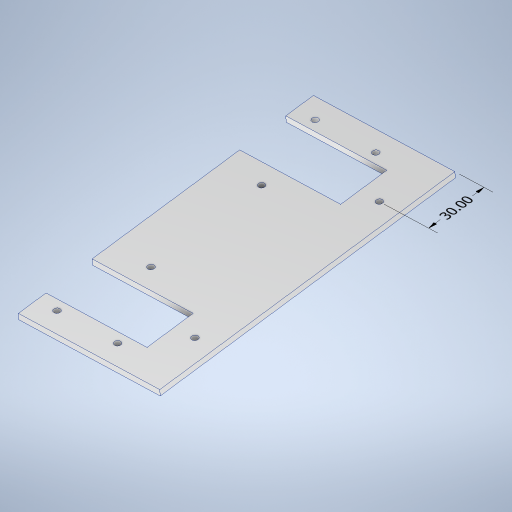
# Autodesk Inventor part: backPlate
Saved by Autodesk Inventor 2024 (Build 280153000, 153)
## iProperties
Created: 2023-10-26
Part Number: backPlate
Material: アルミニウム 6061
Document SubType Name: Modeling
Designer: jwith
Density: 2.7 g/cm^3
Appearance: アルミニウム - フラット
Mass: 69.9488 g
Surface Area: 194.926 cm^2
Volume: 25.907 cm^3
Author: jwith
Autodesk Inventor part; units mm, degrees
ref_plane "YZ Plane" through (0, 0, 0) normal (1, 0, 0) x (0, 1, 0)
ref_plane "XZ Plane" through (0, 0, 0) normal (0, 1, 0) x (-1, 0, 0)
ref_plane "XY Plane" through (0, 0, 0) normal (0, 0, 1) x (1, 0, 0)
sketch "スケッチ1" plane through (0, 0, 0) normal (0, 0, 1) x (1, 0, 0)
  line L0 (0, 0) -> (160, 0)
  line L1 (160, 0) -> (160, 70)
  line L2 (160, 70) -> (0, 70)
  line L3 (0, 70) -> (0, 0)
  line L4 (20, 0) -> (40, 0)
  line L5 (40, 0) -> (40, 50)
  line L6 (40, 50) -> (20, 50)
  line L7 (20, 50) -> (20, 0)
  line L8 (140, 0) -> (120, 0)
  line L9 (120, 0) -> (120, 50)
  line L10 (120, 50) -> (140, 50)
  line L11 (140, 50) -> (140, 0)
  dimension "d0" = 70
  dimension "d1" = 160
  dimension "d2" = 20
  dimension "d3" = 20
  dimension "d4" = 50
  dimension "d5" = 20
  dimension "d6" = 20
  dimension "d7" = 50
  constraints: 24 end point, 6 parallel, 3 horizontal, 3 perpendicular, 2 point on line
  measures "d0" distance of L0.end L1.end
  measures "d1" distance of L1.end L2.end
  measures "d2" distance between parallel lines of L3 L7
  measures "d3" distance of L5.end L6.end
  measures "d4" distance of L4.end L5.end
  measures "d5" distance between parallel lines of L1 L11
  measures "d6" distance of L9.end L10.end
  measures "d7" distance of L10.end L8.start
extrude "押し出し1" add sketch "スケッチ1" along normal blind 3 contours L3 L2 L1 L0 L11 L10 L9 L5 L6 L7
sketch "スケッチ2" plane through (0, 0, 3) normal (0, 0, 1) x (1, 0, 0)
  line L0 (0, 70) -> (0, 0) projected
  line L1 (0, 0) -> (20, 0) projected
  line L2 (140, 0) -> (160, 0) projected
  line L3 (160, 0) -> (160, 70) projected
  point P0 (10, 10)
  point P1 (150, 10)
  point P2 (10, 40)
  point P3 (150, 40)
  dimension "d10" = 10
  dimension "d11" = 10
  dimension "d12" = 10
  dimension "d13" = 10
  dimension "d14" = 30
  dimension "d15" = 10
  dimension "d16" = 10
  dimension "d17" = 30
  measures "d10" distance from line of L0 point (10, 10)
  measures "d11" distance from line of L1 point (10, 10)
  measures "d12" distance from line of L2 point (150, 10)
  measures "d13" distance from line of L3 point (150, 10)
  measures "d14" distance of point (10, 10) point (10, 40)
  measures "d15" distance from line of L0 point (10, 40)
  measures "d16" distance from line of L3 point (150, 40)
  measures "d17" distance of point (150, 10) point (150, 40)
hole "穴1" at (10, 10, 3) at (150, 10, 3) at (10, 40, 3) at (150, 40, 3) direction (0, 0, -1) diameter 3.2 end through all
sketch "スケッチ3" plane through (0, 0, 3) normal (0, 0, 1) x (1, 0, 0)
  line L0 (0, 70) -> (0, 0) projected
  line L1 (160, 70) -> (0, 70) projected
  point P0 (30, 60)
  point P1 (130, 60)
  dimension "d25" = 30
  dimension "d26" = 10
  dimension "d27" = 10
  dimension "d28" = 100
  measures "d25" distance from line of L0 point (30, 60)
  measures "d26" distance from line of L1 point (30, 60)
  measures "d27" distance from line of L1 point (130, 60)
  measures "d28" distance of point (130, 60) point (30, 60)
hole "穴2" at (30, 60, 3) at (130, 60, 3) direction (0, 0, -1) diameter 3.2 end through all
sketch "スケッチ4" plane through (0, 0, 3) normal (0, 0, 1) x (1, 0, 0)
  line L0 (40, 0) -> (120, 0) projected
  line L1 (40, 50) -> (40, 0) projected
  line L2 (120, 0) -> (120, 50) projected
  point P0 (0, 0)
  point P1 (50, 20)
  point P2 (40, 25)
  point P3 (110, 20)
  dimension "d38" = 20
  dimension "d39" = 10
  dimension "d40" = 20
  dimension "d41" = 10
  constraints: 1 midpoint
  measures "d38" distance from line of L0 point (50, 20)
  measures "d39" horizontal distance of point (40, 25) point (50, 20)
  measures "d40" distance from line of L0 point (110, 20)
  measures "d41" distance from line of L2 point (110, 20)
hole "穴3" at (50, 20, 3) at (110, 20, 3) direction (0, 0, -1) diameter 3.2 end through all
sketch "スケッチ5" plane through (0, 0, 3) normal (0, 0, 1) x (1, 0, 0)
  line L0 (20, 0) -> (20, 50) projected
  line L1 (20, 0) -> (15, 0)
  line L2 (15, 0) -> (15, 50)
  line L3 (15, 50) -> (20, 50)
  line L4 (20, 50) -> (20, 0)
  point P0 (0, 0)
  dimension "d49" = 50
  dimension "d50" = 5
  constraints: 8 end point, 2 parallel, 1 horizontal, 1 perpendicular
  measures "d49" distance of L1.end L2.end
  measures "d50" distance between parallel lines of L2 L0
extrude "押し出し2" cut sketch "スケッチ5" against normal blind 3
sketch "スケッチ6" plane through (0, 0, 3) normal (0, 0, 1) x (1, 0, 0)
  line L0 (140, 50) -> (140, 0) projected
  line L1 (140, 0) -> (145, 0)
  line L2 (145, 0) -> (145, 50)
  line L3 (145, 50) -> (140, 50)
  line L4 (140, 50) -> (140, 0)
  point P0 (0, 0)
  dimension "d53" = 50
  dimension "d54" = 5
  constraints: 8 end point, 2 parallel, 1 horizontal, 1 perpendicular
  measures "d53" distance of L1.end L2.end
  measures "d54" distance of L0.end L1.end
extrude "押し出し3" cut sketch "スケッチ6" against normal blind 3
